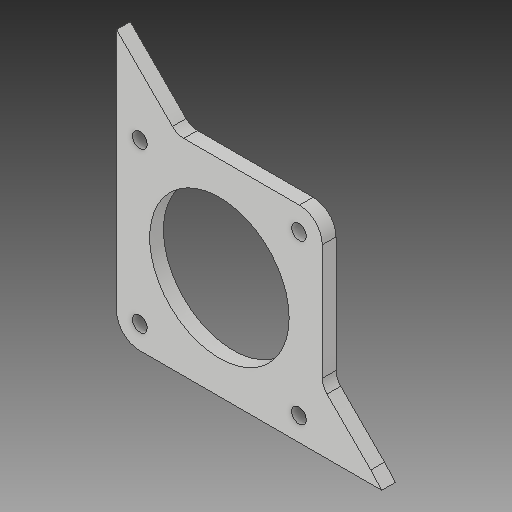
# Autodesk Inventor part: Motor support
Saved by Autodesk Inventor 2018 (Build 220112000, 112)
## iProperties
Created: 2017-06-06
Part Number: Motor support
Material: Generic
Document SubType Name: Modeling
Designer: m228540
Density: 1 g/cm^3
Appearance: Default
Author: m228540
Autodesk Inventor part; units mm, degrees
ref_plane "YZ Plane" through (0, 0, 0) normal (1, 0, 0) x (0, 1, 0)
ref_plane "XZ Plane" through (0, 0, 0) normal (0, 1, 0) x (-1, 0, 0)
ref_plane "XY Plane" through (0, 0, 0) normal (0, 0, 1) x (1, 0, 0)
sketch "Sketch1" plane through (0, 0, 0) normal (0, 0, 1) x (1, 0, 0)
  line L0 (-74.8322, 32.4161) -> (-4.8322, 32.4161)
  line L1 (5.1678, 22.4161) -> (5.1678, -47.5839)
  line L2 (-4.8322, -57.5839) -> (-74.8322, -57.5839)
  line L3 (-84.8322, -47.5839) -> (-84.8322, 22.4161)
  arc A0 (-74.8322, 32.4161) -> (-84.8322, 22.4161) centre (-74.8322, 22.4161) ccw
  arc A1 (5.1678, 22.4161) -> (-4.8322, 32.4161) centre (-4.8322, 22.4161) ccw
  arc A2 (-4.8322, -57.5839) -> (5.1678, -47.5839) centre (-4.8322, -47.5839) ccw
  arc A3 (-84.8322, -47.5839) -> (-74.8322, -57.5839) centre (-74.8322, -47.5839) ccw
  point P0 (0, 0)
  point P1 (-84.8322, 32.4161)
  point P2 (5.1678, 32.4161)
  point P3 (-84.8322, -57.5839)
  dimension "d0" = 90
  dimension "d1" = 90
  dimension "d2" = 10
  constraints: 8 end point, 8 point on circle, 8 tangent, 6 point on line, 4 centre point, 3 equal radius, 2 parallel, 1 horizontal, 1 perpendicular
  measures "d0" distance of point (-84.832, -57.584) point (-84.832, 32.416)
  measures "d1" distance of point (-84.832, 32.416) point (5.168, 32.416)
  measures "d2" radius of A0
extrude "Extrusion1" add sketch "Sketch1" along normal blind 6
sketch "Sketch2" plane through (0, 0, 6) normal (0, 0, 1) x (1, 0, 0)
  line L0 (-84.8322, -47.5839) -> (-84.8322, 22.4161) projected
  line L1 (-84.8322, -12.5839) -> (5.1678, -12.5839) construction
  line L2 (5.1678, 22.4161) -> (5.1678, -47.5839) projected
  circle A0 centre (-39.8322, -12.5839) radius 30.5
  point P0 (0, 0)
  dimension "d5" = 61
  constraints: 3 midpoint, 2 end point, 1 centre point
  measures "d5" diameter of A0
extrude "Extrusion2" cut sketch "Sketch2" against normal through all
sketch "Sketch3" plane through (0, 0, 6) normal (0, 0, 1) x (1, 0, 0)
  line L0 (5.1678, -47.5839) -> (5.1678, 22.4161) projected
  line L1 (5.1678, -12.5839) -> (30.1678, -12.5839) construction
  line L2 (26.381, -52.2971) -> (5.1678, -31.0839)
  circle A0 centre (-39.8322, -12.5839) radius 30.5 projected
  line L3 (-39.8322, -12.5839) -> (-18.2655, 8.9829) construction
  line L4 (-79.5454, 53.6293) -> (-58.3322, 32.4161)
  line L5 (-74.8322, -57.5839) -> (-4.8322, -57.5839) projected
  line L6 (-4.8322, -57.5839) -> (31.1678, -57.5839)
  line L7 (31.1678, -57.5839) -> (26.381, -52.2971)
  arc A1 (-74.8322, 32.4161) -> (-84.8322, 22.4161) centre (-74.8322, 22.4161) ccw projected
  line L8 (-84.8322, 22.4161) -> (-84.8322, 58.9161)
  line L9 (-84.8322, 58.9161) -> (-79.5454, 53.6293)
  line L10 (-4.8322, 32.4161) -> (-74.8322, 32.4161) projected
  line L11 (-58.3322, 32.4161) -> (-74.8322, 32.4161)
  arc A2 (-4.8322, -57.5839) -> (5.1678, -47.5839) centre (-4.8322, -47.5839) ccw projected
  line L12 (5.1678, -31.0839) -> (5.1678, -47.5839)
  point P0 (0, 0)
  dimension "d13" = 53.5
  constraints: 20 end point, 2 horizontal, 2 symmetric about line, 2 tangent, 2 vertical, 1 collinear, 1 midpoint, 1 point on line, 2 other
  measures "d13" distance of L0.end L2.end
extrude "Extrusion3" add sketch "Sketch3" against normal up to surface (6 mm away) contours L0 L2 L7 L6 A2 | L4 L10 A1 L8 L9
fillet "Fillet1" radius 7 2 edges at (-58.3322, 32.4161, 3) (5.1678, -31.0839, 3)
sketch "Sketch4" plane through (0, 0, 0) normal (0, 0, -1) x (-1, 0, 0)
  circle A0 centre (74.6322, 22.2161) radius 3.25 projected
  circle A1 centre (74.6322, -47.3839) radius 3.25 projected
  circle A2 centre (5.0322, -47.3839) radius 3.25 projected
  circle A3 centre (5.0322, 22.2161) radius 3.25 projected
  point P0 (0, 0)
extrude "Extrusion4" cut sketch "Sketch4" against normal through all
body "Solid1"
